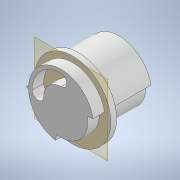
# Autodesk Inventor part: HandleGear2
Saved by Autodesk Inventor 2021 (Build 250183000, 183)
## iProperties
Created: 2021-03-29
Part Number: HandleGear2
Material: Generic
Document SubType Name: Modeling
Designer: ben
Density: 1 g/cm^3
Appearance: Default
Sheet Metal Rule: Default
Author: ben
Autodesk Inventor part; units mm, degrees
ref_plane "YZ Plane" through (0, 0, 0) normal (1, 0, 0) x (0, 1, 0)
ref_plane "XZ Plane" through (0, 0, 0) normal (0, 1, 0) x (-1, 0, 0)
ref_plane "XY Plane" through (0, 0, 0) normal (0, 0, 1) x (1, 0, 0)
sketch "Sketch1" plane through (0, 0, 0) normal (0, 0, 1) x (1, 0, 0)
  circle A0 centre (0.6539, 4.9671) radius 28 projected
  arc A1 (0.5881, 29.9671) -> (-24.346, 4.9013) centre (0.6539, 4.9671) ccw projected
  arc A2 (0.6144, 19.9671) -> (0.5881, 29.9671) centre (0.6013, 24.9671) ccw projected
  arc A3 (0.6144, 19.9671) -> (-14.346, 4.9276) centre (0.6539, 4.9671) ccw projected
  arc A4 (-24.346, 4.9013) -> (-14.346, 4.9276) centre (-19.346, 4.9145) ccw projected
  arc A5 (-3.34, -17.6834) -> (23.3045, 8.961) centre (0.6539, 4.9671) ccw
  line L0 (0.6539, 4.9671) -> (-3.34, -17.6834) construction
  line L1 (0.6539, 4.9671) -> (23.6539, 4.9671) construction
  line L2 (0.6539, 4.9671) -> (23.3045, 8.961) construction
  line L3 (-3.34, -17.6834) -> (-4.2082, -22.6075)
  line L4 (23.3045, 8.961) -> (28.2286, 9.8293)
  line L5 (3.5807, 4.2407) -> (3.5461, 4.234) projected
  line L6 (3.5461, 4.234) -> (-1.7358, 6.7538) projected
  line L7 (-1.7358, 6.7538) -> (-1.7524, 6.7849) projected
  arc A6 (-1.7524, 6.7849) -> (-2.201, 5.8445) centre (0.6899, 5.0426) ccw projected
  line L8 (-2.201, 5.8445) -> (-2.1664, 5.8512) projected
  line L9 (-2.1664, 5.8512) -> (3.1156, 3.3315) projected
  line L10 (3.1156, 3.3315) -> (3.1321, 3.3004) projected
  arc A7 (3.1321, 3.3004) -> (3.5807, 4.2407) centre (0.6899, 5.0426) ccw projected
  line L11 (-2.3009, 4.8074) -> (-1.5498, 5.2584) projected
  line L12 (-1.5498, 5.2584) -> (-2.201, 5.8445) projected
  arc A8 (-2.201, 5.8445) -> (-2.3009, 4.8074) centre (0.6899, 5.0426) ccw projected
  line L13 (-2.0401, 3.7987) -> (-1.4885, 4.4794) projected
  line L14 (-1.4885, 4.4794) -> (-2.3009, 4.8074) projected
  arc A9 (-2.3009, 4.8074) -> (-2.0401, 3.7987) centre (0.6899, 5.0426) ccw projected
  line L15 (-1.45, 2.94) -> (-1.1645, 3.7683) projected
  line L16 (-1.1645, 3.7683) -> (-2.0401, 3.7987) projected
  arc A10 (-2.0401, 3.7987) -> (-1.45, 2.94) centre (0.6899, 5.0426) ccw projected
  line L17 (-1.45, 2.94) -> (-1.1645, 3.7683) projected
  line L18 (-1.1645, 3.7683) -> (-2.0401, 3.7987) projected
  arc A11 (-2.0401, 3.7987) -> (-1.45, 2.94) centre (0.6899, 5.0426) ccw projected
  line L19 (-0.6168, 3.211) -> (-1.45, 2.94) projected
  arc A12 (-1.45, 2.94) -> (-0.6018, 2.335) centre (0.6899, 5.0426) ccw projected
  line L20 (-0.6018, 2.335) -> (-0.6168, 3.211) projected
  line L21 (0.0884, 2.8745) -> (-0.6018, 2.335) projected
  arc A13 (-0.6018, 2.335) -> (0.4021, 2.0565) centre (0.6899, 5.0426) ccw projected
  line L22 (0.4021, 2.0565) -> (0.0884, 2.8745) projected
  line L23 (0.8663, 2.7996) -> (0.4021, 2.0565) projected
  arc A14 (0.4021, 2.0565) -> (1.4408, 2.1381) centre (0.6899, 5.0426) ccw projected
  line L24 (1.4408, 2.1381) -> (0.8663, 2.7996) projected
  line L25 (1.6228, 2.9952) -> (1.4408, 2.1381) projected
  arc A15 (1.4408, 2.1381) -> (2.3889, 2.5701) centre (0.6899, 5.0426) ccw projected
  line L26 (2.3889, 2.5701) -> (1.6228, 2.9952) projected
  line L27 (3.1321, 3.3004) -> (2.2668, 3.4377) projected
  line L28 (2.2668, 3.4377) -> (2.3889, 2.5701) projected
  arc A16 (2.3889, 2.5701) -> (3.1321, 3.3004) centre (0.6899, 5.0426) ccw projected
  line L29 (3.6806, 5.2778) -> (2.9295, 4.8268) projected
  line L30 (2.9295, 4.8268) -> (3.5807, 4.2407) projected
  arc A17 (3.5807, 4.2407) -> (3.6806, 5.2778) centre (0.6899, 5.0426) ccw projected
  line L31 (2.8682, 5.6058) -> (3.6806, 5.2778) projected
  arc A18 (3.6806, 5.2778) -> (3.4198, 6.2865) centre (0.6899, 5.0426) ccw projected
  line L32 (3.4198, 6.2865) -> (2.8682, 5.6058) projected
  line L33 (2.5442, 6.3169) -> (3.4198, 6.2865) projected
  arc A19 (3.4198, 6.2865) -> (2.8297, 7.1452) centre (0.6899, 5.0426) ccw projected
  line L34 (2.8297, 7.1452) -> (2.5442, 6.3169) projected
  line L35 (1.9966, 6.8743) -> (2.8297, 7.1452) projected
  arc A20 (2.8297, 7.1452) -> (1.9816, 7.7503) centre (0.6899, 5.0426) ccw projected
  line L36 (1.9816, 7.7503) -> (1.9966, 6.8743) projected
  line L37 (1.2913, 7.2108) -> (1.9816, 7.7503) projected
  arc A21 (1.9816, 7.7503) -> (0.9776, 8.0288) centre (0.6899, 5.0426) ccw projected
  line L38 (0.9776, 8.0288) -> (1.2913, 7.2108) projected
  line L39 (0.5135, 7.2857) -> (0.9776, 8.0288) projected
  arc A22 (0.9776, 8.0288) -> (-0.0611, 7.9471) centre (0.6899, 5.0426) ccw projected
  line L40 (-0.0611, 7.9471) -> (0.5135, 7.2857) projected
  line L41 (-1.0092, 7.5151) -> (-0.2431, 7.0901) projected
  line L42 (-0.2431, 7.0901) -> (-0.0611, 7.9471) projected
  arc A23 (-0.0611, 7.9471) -> (-1.0092, 7.5151) centre (0.6899, 5.0426) ccw projected
  line L43 (-1.7524, 6.7849) -> (-0.8871, 6.6475) projected
  line L44 (-0.8871, 6.6475) -> (-1.0092, 7.5151) projected
  arc A24 (-1.0092, 7.5151) -> (-1.7524, 6.7849) centre (0.6899, 5.0426) ccw projected
  line L45 (0.6899, 5.0426) -> (-27.346, 5.0426)
  line L46 (-29.346, 5.0426) -> (-26.346, 6.7747)
  line L47 (-26.346, 6.7747) -> (-26.346, 3.3106)
  line L48 (-26.346, 3.3106) -> (-29.346, 5.0426)
  point P0 (0, 0)
  point P1 (-27.3248, 3.8757)
  point P2 (-27.3183, 6.2133)
  point P3 (0.457, 4.0078)
  point P4 (0.4735, 4.5919)
  point P5 (0.5042, 5.6852)
  point P6 (3.4147, 6.0323)
  point P7 (2.8549, 6.911)
  point P8 (2.8549, 6.911)
  point P9 (2.0283, 7.5453)
  point P10 (-1.737, 6.7105)
  point P11 (0.0412, 4.7981)
  point P12 (-0.7372, 6.2774)
  point P13 (-1.737, 6.7105)
  point P14 (-2.2181, 5.7864)
  point P15 (3.4147, 6.0323)
  point P16 (3.6402, 5.0151)
  point P17 (2.0283, 7.5453)
  point P18 (1.48, 2.0033)
  point P19 (0.9312, 4.3735)
  point P20 (0.2466, 4.7001)
  point P21 (1.9636, 4.989)
  point P22 (1.6668, 4.939)
  point P23 (-0.7421, 2.2232)
  point P24 (1.8206, 5.0572)
  point P25 (-0.7421, 2.2232)
  point P26 (0.2515, 1.9099)
  point P27 (0.2515, 1.9099)
  point P28 (1.2924, 1.9553)
  point P29 (1.2924, 1.9553)
  point P30 (2.255, 2.3541)
  point P31 (2.255, 2.3541)
  point P32 (3.0232, 3.058)
  point P33 (3.0232, 3.058)
  point P34 (3.5043, 3.9821)
  point P35 (3.6185, 5.2674)
  point P36 (3.6402, 5.0151)
  point P37 (0.0233, 4.8322)
  point P38 (-0.2672, 4.6867)
  point P39 (3.4147, 6.0323)
  point P40 (-2.3559, 4.806)
  point P41 (-2.1379, 3.7591)
  point P42 (-1.555, 2.8426)
  point P43 (3.6402, 5.0151)
  point P44 (0.4808, 4.8509)
  point P45 (2.9168, 3.4263)
  point P46 (-2.1989, 5.8449)
  point P47 (-0.0075, 4.8213)
  dimension "d8" = 23
  dimension "d9" = 100
  dimension "d10" = 110
  dimension "d11" = 4.924
  dimension "d12" = 4.924
  dimension "d18" = 3
  constraints: 18 end point, 5 point on circle, 2 horizontal, 1 centre point, 1 coincident, 1 equal length, 1 point on line, 7 other
  measures "d8" radius of A5
  measures "d9" angle of L0 L1
  measures "d10" angle of L0 L2
  measures "d11" horizontal distance of L2.end L4.end
  measures "d12" vertical distance of L0.end L3.end
  measures "d18" horizontal distance of L46.start L46.end
ref_plane "Work Plane1" through (-27.427, -23.1101, -9.6285) normal (0, 0, 1) x (0.9999965, 0.0026331, 0)
extrude "Extrusion3" add sketch "Sketch1" along normal blind -35 contours L4 A5 L3 A0 L48 L47 L46 | L46 L47 L45 A0 | A0 L48 L46 | A0 L45 L47 L48 | A7 L10 L9 L8 A6 L7 L6 L5 | L5 L6 L7 L43 L44 L41 L42 L40 L39 L38 L37 L36 L35 L34 L33 L32 L31 L29 L30 | L30 L29 A17 | L27 L28 L26 L25 L24 L23 L22 L21 L20 L19 L15 L16 L13 L14 L11 L45 L9 L10 | A16 L28 L27 | L31 L32 A18 | A15 L25 L26 | L33 L34 A19 | A24 L44 L43 | L45 L11 L12 L8 L9 | A14 L23 L24 | L35 L36 A20 | L12 L11 L45 A8 | A23 L42 L41 | L11 A8 L45 | A13 L21 L22 | L37 L38 A21 | A22 L39 L40 | L14 L13 A9 | A12 L19 L20 | L16 L15 A10
sketch "Sketch6" plane through (0, 0, 0) normal (0, 0, 1) x (-1, 0, 0)
  line L0 (-13, 18) -> (15, 18)
  line L1 (15, 18) -> (15, -27)
  line L2 (15, -27) -> (-13, -27)
  line L3 (-13, -27) -> (-13, 18)
  line L4 (26.346, -3.3106) -> (29.346, -5.0426) projected
  line L5 (29.346, -5.0426) -> (26.346, -6.7747) projected
  arc A0 (4.2082, 22.6075) -> (27.3248, -3.8757) centre (-0.6539, -4.9671) ccw projected
  arc A1 (27.3183, -6.2133) -> (-28.2286, -9.8293) centre (-0.6539, -4.9671) ccw projected
  line L6 (-23.3045, -8.961) -> (-28.2286, -9.8293) projected
  arc A2 (-23.3045, -8.961) -> (3.34, 17.6834) centre (-0.6539, -4.9671) ccw projected
  line L7 (4.2082, 22.6075) -> (3.34, 17.6834) projected
  point P0 (0, 0)
  point P1 (15, -18.2483)
  point P2 (-13, -24.3727)
  dimension "d27" = 28
  dimension "d28" = 45
  constraints: 8 end point, 2 parallel, 1 horizontal, 1 perpendicular
  measures "d27" distance of L1.end L2.end
  measures "d28" distance of L0.end L1.end
extrude "Extrusion6" [suppressed]
sketch "Sketch8" plane through (0, 0, -10) normal (0, 0, -1) x (-1, 0, 0)
  arc A0 (24.346, 4.9013) -> (-0.5881, 29.9671) centre (-0.6539, 4.9671) ccw projected
  arc A1 (15, 2.4422) -> (24.346, 4.9013) centre (19.346, 4.9145) ccw projected
  arc A2 (6.772, 18) -> (-0.6144, 19.9671) centre (-0.6539, 4.9671) ccw projected
  circle A3 centre (19.346, 4.9145) radius 5
  point P0 (0, 0)
  point P1 (16.846, 4.9211)
  point P2 (15, 12.7905)
  point P3 (24.346, 4.9013)
  point P4 (14.346, 4.9276)
  point P5 (24.346, 4.9013)
  point P6 (15, 2.4422)
  constraints: 1 centre point, 1 coincident, 1 concentric
extrude "Extrusion7" [suppressed]
ref_plane "Work Plane2" through (0, 0, -25) normal (0, 0, -1) x (1, 0, 0)
sketch "Sketch9" plane through (0, 0, -25) normal (0, 0, -1) x (1, 0, 0)
  arc A0 (-19.2944, 14.6814) -> (27.4656, -13.0378) centre (0.6539, -4.9671) ccw projected
  arc A1 (-27.3248, -3.8757) -> (-4.2082, 22.6075) centre (0.6539, -4.9671) ccw projected
  arc A2 (27.4656, -13.0378) -> (-19.2944, 14.6814) centre (0.6539, -4.9671) ccw projected
  arc A3 (-31.9701, -9.9343) -> (33.278, -9.9343) centre (0.6539, -4.9671) ccw
  arc A4 (33.278, -9.9343) -> (-31.9701, -9.9343) centre (0.6539, -4.9671) ccw
  point P0 (0, 0)
  dimension "d34" = 5
  constraints: 4 point on circle, 2 centre point, 1 other
  measures "d34" radial gap between concentric circles of A2 A4
extrude "Extrusion8" add sketch "Sketch9" against normal blind 5 contours A2 A1 A0 | A4 A3
equation "\"BendRadius\" = Thickness"
equation "\"BendReliefWidth\" = Thickness"
equation "\"BendReliefDepth\" = 0.5 * Thickness"
equation "\"CornerReliefSize\" = 4 * Thickness"
equation "\"MinimumRemnant\" = 2 * Thickness"
equation "\"TransitionRadius\" = BendRadius"
equation "\"JacobiRadiusSize\" = Thickness"
equation "\"GapSize\" = Thickness"
equation "\"Thickness\" = 0.5"
body "Solid3"
